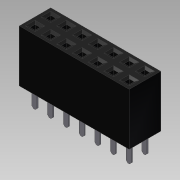
# Autodesk Inventor part: PBD-14
Saved by Autodesk Inventor 2011 (Build 150239000, 239)
## iProperties
Created: 2011-01-10
Part Number: PBD-14
Document SubType Name: Modeling
Designer: abbath
Density: 1 g/cm^3
Author: abbath
Autodesk Inventor part; units mm, degrees
ref_plane "YZ Plane" through (0, 0, 0) normal (1, 0, 0) x (0, 1, 0)
ref_plane "XZ Plane" through (0, 0, 0) normal (0, 1, 0) x (-1, 0, 0)
sketch "Эскиз1" plane through (0, 0, 0) normal (0, 0, 1) x (1, 0, 0)
  line L0 (-8.89, 2.54) -> (8.89, 2.54)
  line L1 (8.89, 2.54) -> (8.89, -2.54)
  line L2 (8.89, -2.54) -> (-8.89, -2.54)
  line L3 (-8.89, -2.54) -> (-8.89, 2.54)
  point P0 (0, 0)
  dimension "d0" = 17.78
  dimension "d1" = 5.08
  dimension "d2" = 8.89
  dimension "d3" = 2.54
  constraints: 8 end point, 2 parallel, 1 horizontal, 1 perpendicular
  measures "d0" distance between parallel lines of L1 L3
  measures "d1" distance between parallel lines of L2 L0
  measures "d2" distance from line of point (0, 0) L3
  measures "d3" distance from line of L0 point (0, 0)
extrude "Выдавливание1" add sketch "Эскиз1" along normal blind 8.4
sketch "Эскиз2" plane through (0, 0, 0) normal (0, 0, -1) x (-1, 0, 0)
  line L0 (-8.89, -2.54) -> (8.89, -2.54) projected
  line L1 (8.89, -2.54) -> (8.89, 2.54) projected
  line L2 (8.02, -1.37) -> (7.22, -1.37)
  line L3 (7.22, -1.37) -> (7.22, -1.17)
  line L4 (7.22, -1.17) -> (8.02, -1.17)
  line L5 (8.02, -1.17) -> (8.02, -1.37)
  line L6 (8.02, -1.27) -> (7.22, -1.27) construction
  line L7 (7.62, -1.37) -> (7.62, -1.17) construction
  point P0 (0, 0)
  dimension "d6" = 0.2
  dimension "d7" = 0.8
  dimension "d8" = 1.27
  dimension "d9" = 1.27
  constraints: 12 end point, 4 midpoint, 2 parallel, 1 horizontal, 1 perpendicular
  measures "d6" distance between parallel lines of L4 L2
  measures "d7" distance between parallel lines of L3 L5
  measures "d8" distance between parallel lines of L1 L7
  measures "d9" distance between parallel lines of L0 L6
extrude "Выдавливание2" add sketch "Эскиз2" along normal blind 3.2
sketch "Эскиз3" plane through (-8.02, -1.37, 0) normal (0, -1, 0) x (1, 0, 0)
  line L0 (0, -3.2) -> (0.8, -3.2) projected
  line L1 (0.8, 0) -> (0.8, -3.2) projected
  line L2 (0, 0) -> (0, -3.2) projected
  line L3 (0, -2.9337) -> (0.2663, -3.2)
  line L4 (0.5326, -3.2) -> (0.8, -2.9326)
  point P0 (8.02, 0)
  dimension "d14" = 45
  dimension "d15" = 0.2663
  dimension "d16" = 0.2663
  constraints: 4 end point, 4 point on line, 1 perpendicular
  measures "d14" angle of L3 L0
  measures "d15" distance from line of L3.end L2
  measures "d16" distance of L4.start L3.end
extrude "Выдавливание3" cut sketch "Эскиз3" against normal through all
pattern_linear "Прямоуг.массив1" count 7 spacing 2.54 along (1, 0, 0) count 2 spacing 2.54 along (0, 1, 0) of "Выдавливание3", "Выдавливание2"
sketch "Эскиз4" plane through (0, 0, 8.4) normal (0, 0, 1) x (1, 0, 0)
  line L0 (-7.4874, -1.17) -> (-7.4874, -1.37) projected
  line L1 (-7.7537, -1.37) -> (-7.4874, -1.37) projected
  line L2 (-7.7537, -1.37) -> (-7.7537, -1.17) projected
  line L3 (-7.4874, -1.17) -> (-7.7537, -1.17) projected
  line L4 (-8.4206, -0.47) -> (-6.8206, -0.47)
  line L5 (-6.8206, -0.47) -> (-6.8206, -2.07)
  line L6 (-6.8206, -2.07) -> (-8.4206, -2.07)
  line L7 (-8.4206, -2.07) -> (-8.4206, -0.47)
  point P0 (0, 0)
  dimension "d25" = 0.7
  dimension "d26" = 1.6
  dimension "d27" = 0.7
  dimension "d28" = 0.6669
  dimension "d29" = 1.6
  dimension "d30" = 0.6669
  constraints: 8 end point, 2 parallel, 1 horizontal, 1 perpendicular
  measures "d25" distance between parallel lines of L3 L4
  measures "d26" distance between parallel lines of L6 L4
  measures "d27" distance between parallel lines of L1 L6
  measures "d28" distance between parallel lines of L2 L7
  measures "d29" distance between parallel lines of L5 L7
  measures "d30" distance between parallel lines of L5 L0
ref_plane "РабПлоскость1" through (0, 0, 8.2) normal (0, 0, 1) x (1, 0, 0)
sketch "Эскиз5" plane through (0, 0, 8.2) normal (0, 0, 1) x (1, 0, 0)
  line L0 (-8.4206, -2.07) -> (-8.4206, -0.47) projected
  line L1 (-8.4206, -0.47) -> (-6.8206, -0.47) projected
  line L2 (-6.8206, -0.47) -> (-6.8206, -2.07) projected
  line L3 (-6.8206, -2.07) -> (-8.4206, -2.07) projected
  line L4 (-7.2206, -0.87) -> (-8.0206, -0.87)
  line L5 (-8.0206, -0.87) -> (-8.0206, -1.67)
  line L6 (-8.0206, -1.67) -> (-7.2206, -1.67)
  line L7 (-7.2206, -1.67) -> (-7.2206, -0.87)
  point P0 (0, 0)
  dimension "d32" = 0.8
  constraints: 8 end point, 3 other
  measures "d32" distance between parallel lines of L6 L4
loft "По сечениям1" cut profiles "Эскиз4", "Эскиз5" contours L0 L1 L2 L3 | L4 L5 L6 L7 / L7 L6 L5 L4
sketch "Эскиз6" plane through (-8.0206, -0.87, 8.2) normal (0, 0, 1) x (1, 0, 0)
  line L0 (0, 0) -> (0.8, 0) projected
  line L1 (0, -0.8) -> (0, 0) projected
  line L2 (0.8, -0.8) -> (0, -0.8) projected
  line L3 (0.8, 0) -> (0.8, -0.8) projected
  point P0 (8.0206, 0.87)
extrude "Выдавливание4" cut sketch "Эскиз6" against normal blind 6
pattern_linear "Прямоуг.массив2" count 7 spacing 2.54 along (1, 0, 0) count 2 spacing 2.54 along (0, 1, 0) of "Выдавливание4", "По сечениям1"
equation "\"d2\" = 0.5 * d0"
equation "\"d3\" = 0.5 * d1"
equation "\"d16\" = d15"
equation "\"d25\" = d27"
equation "\"d28\" = d30"
